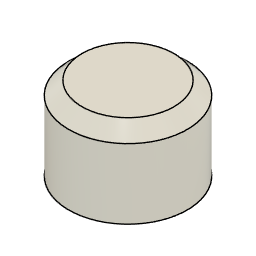
Peg (Single) (Autodesk Fusion 360 design; units mm, degrees)
Autodesk Fusion 360 part; units mm, degrees
sketch "Sketch1" plane through (0, 0, 0) normal (0, 1, 0) x (1, 0, 0)
  circle A0 centre (0, 0) radius 5.715
  dimension "d3" = 11.43
  constraint coincident A0.centre origin
  measures "d3" diameter of A0
extrude "Extrude1" add sketch "Sketch1" along normal blind 8.001 makes body 1
chamfer "Chamfer1" distance 1.27 angle 45 1 edges at (-5.3283, 8.001, 2.0666) on bodies 1
copy_body "Body->Comp1" bodies 1 removing the originals makes body 2 in component "Peg"
component "Peg" placed x (1, 0, 0) y (0, 1, 0) z (0, 0, 1) at (0, 0, 0)
equation "pegDiameter = 0.45 in"
equation "pegDepth = 0.2 in + boardThickness"
equation "d3 = pegDiameter"
equation "d4 = pegDepth"
equation "boardThickness = 0.115 in"
named bodies: "Peg"
